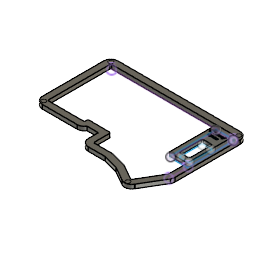
left_top_cover (Autodesk Fusion 360 design; units mm, degrees)
part number: 2026-07-17-00-49-13-895
Autodesk Fusion 360 part; units mm, degrees
note: some values were not read from the file. Set by a fixed rule: which sketch regions a step uses.
sketch "topcoverout1" plane through (0, 0, 0) normal (0, 0, 1) x (1, 0, 0)
  arc A0 (-38.1199, -35.6191) -> (-38.1206, -35.6555) centre (-37.1206, -35.6574) ccw
  line L0 (-38.1206, -35.6555) -> (-38.1199, -35.2716)
  line L1 (-38.1199, -35.2716) -> (-38.1199, -35.6191)
  line L2 (-63.0386, 17.2914) -> (-60.9186, 17.2914)
  line L3 (-72.6386, 3.6665) -> (-74.7361, 3.6665)
  line L4 (-60.941, 3.6665) -> (-63.0386, 3.6665)
  line L5 (-60.9226, 17.2877) -> (-60.9226, 13.2151)
  line L6 (-60.9226, 7.4151) -> (-60.9226, 3.6437)
  line L7 (-74.7546, 3.6437) -> (-74.7546, 7.4151)
  line L8 (-60.8212, 3.327) -> (-74.8212, 3.327)
  line L9 (-60.8212, 17.327) -> (-60.8212, 3.327)
  line L10 (-74.8212, 17.327) -> (-60.8212, 17.327)
  line L11 (-74.8212, 3.327) -> (-74.8212, 17.327)
  line L12 (-74.8212, 17.327) -> (-60.8212, 17.327)
  line L13 (-74.8212, 3.327) -> (-74.8212, 17.327)
  line L14 (-60.8681, -1.6074) -> (-60.8681, -15.6074)
  line L15 (-74.8681, -1.6074) -> (-60.8681, -1.6074)
  line L16 (-60.8681, -15.6074) -> (-74.8681, -15.6074)
  line L17 (-74.8681, -15.6074) -> (-74.8681, -1.6074)
  line L18 (-60.8756, -20.5875) -> (-60.8756, -34.5875)
  line L19 (-74.8756, -20.5875) -> (-60.8756, -20.5875)
  line L20 (-60.8756, -34.5875) -> (-74.8756, -34.5875)
  line L21 (-74.8756, -34.5875) -> (-74.8756, -20.5875)
  line L22 (-74.8618, 3.6522) -> (-74.8618, 17.6522)
  line L23 (-41.7744, 17.3824) -> (-41.7744, 3.3824)
  line L24 (-55.7744, 17.3824) -> (-41.7744, 17.3824)
  line L25 (-41.7744, 3.3824) -> (-55.7744, 3.3824)
  line L26 (-55.7744, 3.3824) -> (-55.7744, 17.3824)
  line L27 (-41.7619, -1.6704) -> (-41.7619, -15.6704)
  line L28 (-55.7619, -1.6704) -> (-41.7619, -1.6704)
  line L29 (-41.7619, -15.6704) -> (-55.7619, -15.6704)
  line L30 (-55.7619, -15.6704) -> (-55.7619, -1.6704)
  line L31 (-41.7679, -20.6705) -> (-41.7679, -34.6705)
  line L32 (-55.7679, -20.6705) -> (-41.7679, -20.6705)
  line L33 (-41.7679, -34.6705) -> (-55.7679, -34.6705)
  line L34 (-55.7679, -34.6705) -> (-55.7679, -20.6705)
  line L35 (-22.6973, 21.268) -> (-22.6973, 7.268)
  line L36 (-36.6973, 21.268) -> (-22.6973, 21.268)
  line L37 (-22.6973, 7.268) -> (-36.6973, 7.268)
  line L38 (-36.6973, 7.268) -> (-36.6973, 21.268)
  line L39 (-22.6915, 2.1961) -> (-22.6915, -11.8039)
  line L40 (-36.6915, 2.1961) -> (-22.6915, 2.1961)
  line L41 (-22.6915, -11.8039) -> (-36.6915, -11.8039)
  line L42 (-36.6915, -11.8039) -> (-36.6915, 2.1961)
  line L43 (44.6185, 10.2372) -> (44.6185, -15.5628)
  line L44 (55.9185, 10.2372) -> (44.6185, 10.2372)
  line L45 (44.6185, -15.5628) -> (55.9185, -15.5628)
  line L46 (55.9185, -15.5628) -> (55.9185, 10.2372)
  line L47 (-22.7318, -16.9097) -> (-22.7318, -30.9097)
  line L48 (-36.7318, -16.9097) -> (-22.7318, -16.9097)
  line L49 (-22.7318, -30.9097) -> (-36.7318, -30.9097)
  line L50 (-36.7318, -30.9097) -> (-36.7318, -16.9097)
  line L51 (-3.7525, 23.0596) -> (-3.7525, 9.0596)
  line L52 (-17.7525, 23.0596) -> (-3.7525, 23.0596)
  line L53 (-3.7525, 9.0596) -> (-17.7525, 9.0596)
  line L54 (-17.7525, 9.0596) -> (-17.7525, 23.0596)
  line L55 (-3.7007, 3.9637) -> (-3.7007, -10.0363)
  line L56 (-17.7007, 3.9637) -> (-3.7007, 3.9637)
  line L57 (-3.7007, -10.0363) -> (-17.7007, -10.0363)
  line L58 (-17.7007, -10.0363) -> (-17.7007, 3.9637)
  line L59 (-3.7688, -15.0165) -> (-3.7688, -29.0165)
  line L60 (-17.7688, -15.0165) -> (-3.7688, -15.0165)
  line L61 (-3.7688, -29.0165) -> (-17.7688, -29.0165)
  line L62 (-17.7688, -29.0165) -> (-17.7688, -15.0165)
  line L63 (15.4185, 21.139) -> (15.4185, 7.139)
  line L64 (1.4185, 21.139) -> (15.4185, 21.139)
  line L65 (15.4185, 7.139) -> (1.4185, 7.139)
  line L66 (1.4185, 7.139) -> (1.4185, 21.139)
  line L67 (15.4509, 2.0912) -> (15.4509, -11.9088)
  line L68 (1.4509, 2.0912) -> (15.4509, 2.0912)
  line L69 (15.4509, -11.9088) -> (1.4509, -11.9088)
  line L70 (1.4509, -11.9088) -> (1.4509, 2.0912)
  line L71 (15.4192, -16.9262) -> (15.4192, -30.9262)
  line L72 (1.4192, -16.9262) -> (15.4192, -16.9262)
  line L73 (15.4192, -30.9262) -> (1.4192, -30.9262)
  line L74 (1.4192, -30.9262) -> (1.4192, -16.9262)
  line L75 (34.4618, 19.276) -> (34.4618, 5.276)
  line L76 (20.4618, 19.276) -> (34.4618, 19.276)
  line L77 (34.4618, 5.276) -> (20.4618, 5.276)
  line L78 (20.4618, 5.276) -> (20.4618, 19.276)
  line L79 (34.3662, 0.0812) -> (34.3662, -13.9188)
  line L80 (20.3662, 0.0812) -> (34.3662, 0.0812)
  line L81 (34.3662, -13.9188) -> (20.3662, -13.9188)
  line L82 (20.3662, -13.9188) -> (20.3662, 0.0812)
  line L83 (34.4383, -18.8384) -> (34.4383, -32.8384)
  line L84 (20.4383, -18.8384) -> (34.4383, -18.8384)
  line L85 (34.4383, -32.8384) -> (20.4383, -32.8384)
  line L86 (20.4383, -32.8384) -> (20.4383, -18.8384)
  line L87 (5.8139, -35.9431) -> (5.8139, -49.9431)
  line L88 (-8.1861, -35.9431) -> (5.8139, -35.9431)
  line L89 (5.8139, -49.9431) -> (-8.1861, -49.9431)
  line L90 (-8.1861, -49.9431) -> (-8.1861, -35.9431)
  line L91 (28.7862, -40.8277) -> (25.1627, -54.3507)
  line L92 (15.2632, -37.2043) -> (28.7862, -40.8277)
  line L93 (25.1627, -54.3507) -> (11.6397, -50.7272)
  line L94 (11.6397, -50.7272) -> (15.2632, -37.2043)
  line L95 (51.7903, -47.2432) -> (44.7903, -59.3676)
  line L96 (39.666, -40.2432) -> (51.7903, -47.2432)
  line L97 (44.7903, -59.3676) -> (32.666, -52.3676)
  line L98 (32.666, -52.3676) -> (39.666, -40.2432)
  line L99 (39.9616, -20.2716) -> (39.9616, 29.8284)
  line L100 (39.9616, 29.8284) -> (59.3616, 29.8284)
  line L101 (59.3616, -20.2716) -> (39.9616, -20.2716)
  line L102 (59.3616, 29.8284) -> (59.3616, -20.2716)
  circle A1 centre (-81.2782, 34.061) radius 1.6
  circle A2 centre (-81.0384, -41.2716) radius 1.6
  circle A3 centre (43.9616, -72.2716) radius 1.6
  circle A4 centre (61.4616, 34.2284) radius 1.6
  line L103 (-37.1187, -34.6575) -> (-37.1033, -34.6575)
  line L104 (-37.1033, -34.6575) -> (-13.5537, -34.8219)
  arc A5 (-12.5607, -35.8288) -> (-13.5537, -34.8219) centre (-13.5606, -35.8219) ccw
  line L105 (-12.5607, -35.8288) -> (-12.5617, -35.9723)
  line L106 (-12.5617, -35.9723) -> (-12.558, -53.0098)
  arc A6 (-12.558, -53.0098) -> (-11.558, -54.0096) centre (-11.558, -53.0096) ccw
  line L107 (-11.558, -54.0096) -> (8.2128, -54.0096)
  arc A7 (8.4715, -54.0436) -> (8.2128, -54.0096) centre (8.2128, -55.0096) ccw
  line L108 (8.4715, -54.0436) -> (26.4518, -58.8585)
  arc A8 (26.6903, -58.9568) -> (26.4518, -58.8585) centre (26.1932, -59.8244) ccw
  line L109 (26.6903, -58.9568) -> (43.1014, -68.3607)
  arc A9 (43.1014, -68.3607) -> (44.4663, -67.9902) centre (43.5986, -67.4931) ccw
  line L110 (44.4663, -67.9902) -> (44.7236, -67.5412)
  line L111 (44.7236, -67.5412) -> (59.4411, -42.5979)
  arc A10 (59.4411, -42.5979) -> (59.5798, -42.0897) centre (58.5798, -42.0897) ccw
  line L112 (59.5798, -42.0897) -> (59.5798, 30.7287)
  arc A11 (59.5798, 30.7287) -> (58.5802, 31.7287) centre (58.5798, 30.7287) ccw
  line L113 (58.5802, 31.7287) -> (-78.1023, 31.7808)
  arc A12 (-78.1023, 31.7808) -> (-79.1027, 30.7808) centre (-78.1027, 30.7808) ccw
  line L114 (-79.1027, 30.7808) -> (-79.1027, -37.7188)
  arc A13 (-79.1027, -37.7188) -> (-78.1027, -38.7188) centre (-78.1027, -37.7188) ccw
  line L115 (-78.1027, -38.7188) -> (-39.1199, -38.7188)
  arc A14 (-39.1199, -38.7188) -> (-38.1199, -37.7188) centre (-39.1199, -37.7188) ccw
  line L116 (-38.1199, -37.7188) -> (-38.1199, -35.6191)
  arc A15 (-37.1187, -34.6575) -> (-38.1199, -35.6191) centre (-37.1206, -35.6574) ccw
  arc A16 (-19.558, -53.0113) -> (-11.558, -61.0096) centre (-11.558, -53.0096) ccw
  line L117 (-19.5604, -41.7801) -> (-19.558, -53.0113)
  line L118 (-86.1027, 30.7808) -> (-86.1027, 27.7812)
  arc A17 (65.4699, -46.1551) -> (66.5798, -42.0897) centre (58.5798, -42.0897) ccw
  line L119 (-7.292, -61.0096) -> (7.4234, -61.0096)
  arc A18 (-86.1027, -37.7188) -> (-78.1027, -45.7188) centre (-78.1027, -37.7188) ccw
  arc A19 (66.5798, 30.7287) -> (58.5829, 38.7287) centre (58.5798, 30.7287) ccw
  line L120 (50.775, -71.06) -> (53.5624, -66.336)
  line L121 (-32.1763, -41.692) -> (-19.5604, -41.7801)
  line L122 (-71.0384, -45.7188) -> (-39.1199, -45.7188)
  arc A20 (39.6212, -74.4342) -> (50.5398, -71.4705) centre (43.5986, -67.4931) ccw
  line L123 (-78.1027, -45.7188) -> (-71.0384, -45.7188)
  line L124 (7.4234, -61.0096) -> (23.8872, -65.4183)
  line L125 (50.5398, -71.4705) -> (50.775, -71.06)
  line L126 (39.4454, -74.3335) -> (39.6212, -74.4342)
  line L127 (58.5829, 38.7287) -> (-78.0996, 38.7808)
  line L128 (23.8872, -65.4183) -> (39.4454, -74.3335)
  arc A21 (-39.1199, -45.7188) -> (-32.1763, -41.692) centre (-39.1199, -37.7188) ccw
  line L129 (53.5624, -66.336) -> (58.9899, -57.1374)
  line L130 (66.5798, -42.0897) -> (66.5798, 30.7287)
  line L131 (-11.558, -61.0096) -> (-7.292, -61.0096)
  line L132 (58.9899, -57.1374) -> (64.9753, -46.9933)
  line L133 (-86.1027, 27.7812) -> (-86.1027, -37.7188)
  line L134 (64.9753, -46.9933) -> (65.4699, -46.1551)
  arc A22 (-78.0996, 38.7808) -> (-86.1027, 30.7808) centre (-78.1027, 30.7808) ccw
  point P0 (61.4616, 34.2284)
  point P1 (-81.2782, 34.061)
  point P2 (-81.0384, -41.2716)
  point P3 (43.9616, -72.2716)
sketch "Sketch2" plane through (0, 0, 0) normal (0, 0, 1) x (1, 0, 0)
  line L0 (39.9616, 29.8284) -> (59.3616, 29.8284)
  line L1 (39.9616, -20.2716) -> (39.9616, 29.8284)
  line L2 (59.3616, -20.2716) -> (39.9616, -20.2716)
  line L3 (58.5802, 31.7287) -> (-78.1023, 31.7808)
  arc A0 (59.5798, 30.7287) -> (58.5802, 31.7287) centre (58.5798, 30.7287) ccw
  line L4 (59.5798, -42.0897) -> (59.5798, 30.7287)
  line L5 (38.6875, 31.7363) -> (58.5798, 31.7363)
  line L6 (59.5798, 30.7363) -> (59.5798, -21.2716)
  line L7 (59.5798, -21.2716) -> (39.6875, -21.2716)
  line L8 (38.6875, -20.2716) -> (38.6875, 31.7363)
  arc A1 (59.5798, 30.7363) -> (58.5798, 31.7363) centre (58.5798, 30.7363) ccw
  arc A2 (38.6875, -20.2716) -> (39.6875, -21.2716) centre (39.6875, -20.2716) ccw
  line L9 (45.6185, 10.2372) -> (54.9185, 10.2372)
  line L10 (55.9185, 9.2372) -> (55.9185, -14.5628)
  line L11 (54.9185, -15.5628) -> (45.6185, -15.5628)
  line L12 (44.6185, -14.5628) -> (44.6185, 9.2372)
  arc A3 (45.6185, 10.2372) -> (44.6185, 9.2372) centre (45.6185, 9.2372) ccw
  arc A4 (55.9185, 9.2372) -> (54.9185, 10.2372) centre (54.9185, 9.2372) ccw
  arc A5 (54.9185, -15.5628) -> (55.9185, -14.5628) centre (54.9185, -14.5628) ccw
  arc A6 (44.6185, -14.5628) -> (45.6185, -15.5628) centre (45.6185, -14.5628) ccw
  dimension "d3" = 1
  dimension "d4" = 1
  dimension "d5" = 1
  constraint perpendicular L5 L6
  constraint parallel L5 L7
  constraint parallel L6 L8
  constraint perpendicular L4 L5
  constraint coincident L3 L5.start
  constraint tangent L5 A1
  constraint tangent L6 A1
  constraint tangent L7 A2
  constraint tangent L8 A2
  constraint perpendicular L9 L10
  constraint parallel L9 L11
  constraint parallel L10 L12
  constraint tangent L9 A3
  constraint tangent L12 A3
  constraint tangent L9 A4
  constraint tangent L10 A4
  constraint equal A3 A4
  constraint tangent L10 A5
  constraint tangent L11 A5
  constraint equal A3 A5
  constraint tangent L11 A6
  constraint tangent L12 A6
  constraint equal A3 A6
  measures "d3" radius of A1
  measures "d4" radius of A2
  measures "d5" radius of A3
extrude "Extrude1" add sketch "topcoverout1" along normal blind 4.5 contours A1 | A2 | A3 | A4 | A16 L117 L118 A17 L119 A18 A19 L120 L121 L122 A20 L123 L124 L125 L126 L127 L128 A21 L129 L130 L131 L132 L133 L134 A22 picked at (-81.0115, 33.1363) picked at (-80.7717, -42.1963) picked at (43.6291, -73.003) picked at (61.7283, 35.0046) picked at (13.0203, 34.0794) makes body 1
extrude "Extrude2" add sketch "Sketch2" along normal blind 4.5 separate body contours L3 A0 L4 L6 L7 L8 A2 picked at (47.6287, 24.5674) makes body 2
sketch "Sketch3" plane through (0, 0, 0) normal (0, 0, 1) x (1, 0, 0)
  circle A0 centre (61.4616, 34.2284) radius 1.6
  circle A1 centre (43.9616, -72.2716) radius 1.6
  circle A2 centre (-81.2782, 34.061) radius 1.6
  circle A3 centre (61.4616, 34.2284) radius 2.45
  circle A4 centre (43.9616, -72.2716) radius 2.45
  circle A5 centre (-81.0384, -41.2716) radius 2.45
  circle A6 centre (-81.2782, 34.061) radius 2.45
  point P0 (-81.0384, -41.2716)
  dimension "d8" = 4.9
  dimension "d9" = 4.9
  dimension "d10" = 4.9
  dimension "d11" = 4.9
  constraint concentric A0 A3
  constraint concentric A1 A4
  constraint coincident P0 A5.centre
  constraint concentric A2 A6
  measures "d8" diameter of A3
  measures "d9" diameter of A4
  measures "d10" diameter of A5
  measures "d11" diameter of A6
extrude "Extrude3" cut sketch "Sketch3" along normal blind 3.9 contours A0 | A1 | A2 | A3 | A4 | A6 picked at (61.7283, 35.0046) picked at (43.6291, -73.003) picked at (-81.0115, 33.1363) picked at (59.3463, 34.6703) picked at (45.8128, -73.3865) picked at (-80.9955, 36.2034) bodies 1
extrude "Extrude4" cut sketch "Sketch3" along normal blind 3.9 contours A5 picked at (-79.2238, -40.9981) bodies 1
extrude "Extrude5" cut 1 faces at (47.6287, 24.5674, 0) along direction (0, 0, 1) blind 0.5 on bodies 2 bodies 2
extrude "Extrude6" cut 1 faces at (47.6287, 24.5674, 0.5) along direction (0, 0, 1) blind 0.5 on bodies 2 bodies 2
sketch "Sketch4" plane through (0, 0, 4.5) normal (0, 0, 1) x (-1, 0, 0)
  arc A0 (-45.6185, -10.2372) -> (-44.6185, -9.2372) centre (-45.6185, -9.2372) ccw
  line L0 (-45.6185, -10.2372) -> (-54.9185, -10.2372)
  arc A1 (-55.9185, -9.2372) -> (-54.9185, -10.2372) centre (-54.9185, -9.2372) ccw
  line L1 (-55.9185, -9.2372) -> (-55.9185, 14.5628)
  arc A2 (-54.9185, 15.5628) -> (-55.9185, 14.5628) centre (-54.9185, 14.5628) ccw
  line L2 (-54.9185, 15.5628) -> (-45.6185, 15.5628)
  arc A3 (-44.6185, 14.5628) -> (-45.6185, 15.5628) centre (-45.6185, 14.5628) ccw
  line L3 (-44.6185, 14.5628) -> (-44.6185, -9.2372)
  arc A4 (-59.5798, -30.7287) -> (-58.5802, -31.7287) centre (-58.5798, -30.7287) ccw
  line L4 (-58.5802, -31.7287) -> (-38.6875, -31.7363)
  line L5 (-38.6875, -31.7363) -> (-38.6875, 20.2716)
  arc A5 (-38.6875, 20.2716) -> (-39.6875, 21.2716) centre (-39.6875, 20.2716) ccw
  line L6 (-39.6875, 21.2716) -> (-59.5798, 21.2716)
  line L7 (-59.5798, 21.2716) -> (-59.5798, -30.7287)
  spline S0 degree 2 poles (-41.2211, -21.734) (-40.7461, -21.7358) (-40.5191, -21.9812) knots 0 0 0 1 1 1
  spline S1 degree 2 poles (-40.5191, -21.9812) (-40.2922, -22.2266) (-40.2904, -22.7615) knots 0 0 0 1 1 1
  spline S2 degree 2 poles (-40.2904, -22.7615) (-40.2922, -23.1837) (-40.3872, -23.5435) knots 0 0 0 1 1 1
  spline S3 degree 2 poles (-40.3872, -23.5435) (-40.4822, -23.9033) (-40.6564, -24.1707) knots 0 0 0 1 1 1
  spline S4 degree 2 poles (-40.6564, -24.1707) (-40.8305, -24.4381) (-41.0628, -24.5868) knots 0 0 0 1 1 1
  spline S5 degree 2 poles (-41.0628, -24.5868) (-41.295, -24.7354) (-41.5677, -24.7354) knots 0 0 0 1 1 1
  spline S6 degree 2 poles (-41.5677, -24.7354) (-42.2046, -24.7354) (-42.2046, -24.0827) knots 0 0 0 1 1 1
  spline S7 degree 2 poles (-42.2046, -24.0827) (-42.2063, -23.9807) (-42.1703, -23.766) knots 0 0 0 1 1 1
  spline S8 degree 2 poles (-42.1703, -23.766) (-42.1342, -23.5514) (-42.0585, -23.1256) knots 0 0 0 1 1 1
  line L8 (-42.0585, -23.1256) -> (-41.6891, -23.1256)
  spline S9 degree 2 poles (-41.6891, -23.1256) (-41.7295, -23.3667) (-41.7542, -23.5215) knots 0 0 0 1 1 1
  spline S10 degree 2 poles (-41.7542, -23.5215) (-41.7788, -23.6763) (-41.7911, -23.7678) knots 0 0 0 1 1 1
  spline S11 degree 2 poles (-41.7911, -23.7678) (-41.8034, -23.8593) (-41.8096, -23.9112) knots 0 0 0 1 1 1
  spline S12 degree 2 poles (-41.8096, -23.9112) (-41.8158, -23.9631) (-41.8228, -23.9965) knots 0 0 0 1 1 1
  spline S13 degree 2 poles (-41.8228, -23.9965) (-41.8245, -24.2094) (-41.7463, -24.2824) knots 0 0 0 1 1 1
  spline S14 degree 2 poles (-41.7463, -24.2824) (-41.668, -24.3554) (-41.5149, -24.3554) knots 0 0 0 1 1 1
  spline S15 degree 2 poles (-41.5149, -24.3554) (-41.3407, -24.3572) (-41.1877, -24.2323) knots 0 0 0 1 1 1
  spline S16 degree 2 poles (-41.1877, -24.2323) (-41.0346, -24.1073) (-40.9176, -23.8892) knots 0 0 0 1 1 1
  spline S17 degree 2 poles (-40.9176, -23.8892) (-40.8006, -23.671) (-40.7338, -23.3843) knots 0 0 0 1 1 1
  spline S18 degree 2 poles (-40.7338, -23.3843) (-40.6669, -23.0975) (-40.6687, -22.772) knots 0 0 0 1 1 1
  spline S19 degree 2 poles (-40.6687, -22.772) (-40.6687, -22.4307) (-40.805, -22.2715) knots 0 0 0 1 1 1
  spline S20 degree 2 poles (-40.805, -22.2715) (-40.9414, -22.1123) (-41.2246, -22.114) knots 0 0 0 1 1 1
  spline S21 degree 2 poles (-41.2246, -22.114) (-41.4498, -22.114) (-41.587, -22.1562) knots 0 0 0 1 1 1
  line L9 (-41.587, -22.1562) -> (-41.5343, -21.778)
  spline S22 degree 2 poles (-41.5343, -21.778) (-41.4023, -21.7358) (-41.2211, -21.734) knots 0 0 0 1 1 1
  spline S23 degree 2 poles (-41.2123, -22.4395) (-41.0557, -22.4395) (-40.9704, -22.5688) knots 0 0 0 1 1 1
  spline S24 degree 2 poles (-40.9704, -22.5688) (-40.8851, -22.6981) (-40.8851, -22.9304) knots 0 0 0 1 1 1
  spline S25 degree 2 poles (-40.8851, -22.9304) (-40.8851, -23.2646) (-41.0117, -23.5188) knots 0 0 0 1 1 1
  spline S26 degree 2 poles (-41.0117, -23.5188) (-41.1384, -23.7731) (-41.3592, -23.9296) knots 0 0 0 1 1 1
  spline S27 degree 2 poles (-41.3592, -23.9296) (-41.58, -24.0862) (-41.8615, -24.1214) knots 0 0 0 1 1 1
  line L10 (-41.8615, -24.1214) -> (-41.8386, -23.7396)
  spline S28 degree 2 poles (-41.8386, -23.7396) (-41.6715, -23.7326) (-41.5351, -23.635) knots 0 0 0 1 1 1
  spline S29 degree 2 poles (-41.5351, -23.635) (-41.3988, -23.5373) (-41.3196, -23.3755) knots 0 0 0 1 1 1
  spline S30 degree 2 poles (-41.3196, -23.3755) (-41.2405, -23.2136) (-41.2405, -23.0095) knots 0 0 0 1 1 1
  spline S31 degree 2 poles (-41.2405, -23.0095) (-41.2405, -22.9057) (-41.2774, -22.8529) knots 0 0 0 1 1 1
  spline S32 degree 2 poles (-41.2774, -22.8529) (-41.3143, -22.8002) (-41.3865, -22.8002) knots 0 0 0 1 1 1
  spline S33 degree 2 poles (-41.3865, -22.8002) (-41.4674, -22.8002) (-41.5307, -22.8609) knots 0 0 0 1 1 1
  spline S34 degree 2 poles (-41.5307, -22.8609) (-41.5941, -22.9216) (-41.6469, -23.0641) knots 0 0 0 1 1 1
  spline S35 degree 2 poles (-41.6469, -23.0641) (-41.6996, -23.2066) (-41.7454, -23.4529) knots 0 0 0 1 1 1
  line L11 (-41.7454, -23.4529) -> (-42.1166, -23.4529)
  line L12 (-42.1166, -23.4529) -> (-41.9442, -22.4729)
  line L13 (-41.9442, -22.4729) -> (-41.6152, -22.4729)
  line L14 (-41.6152, -22.4729) -> (-41.6697, -23.0236)
  line L15 (-41.6697, -23.0236) -> (-41.7718, -22.8477)
  line L16 (-41.7718, -22.8477) -> (-41.5765, -22.8459)
  line L17 (-41.5765, -22.8459) -> (-41.6398, -22.9409)
  spline S36 degree 2 poles (-41.6398, -22.9409) (-41.587, -22.7034) (-41.4736, -22.5723) knots 0 0 0 1 1 1
  spline S37 degree 2 poles (-41.4736, -22.5723) (-41.3601, -22.4413) (-41.2123, -22.4395) knots 0 0 0 1 1 1
  line L18 (-42.9452, -22.2037) -> (-43.1282, -23.2488)
  line L19 (-43.1282, -23.2488) -> (-43.5575, -23.2488)
  line L20 (-43.5575, -23.2488) -> (-43.3745, -22.2037)
  line L21 (-43.3745, -22.2037) -> (-42.9452, -22.2037)
  line L22 (-43.1106, -22.9708) -> (-42.5652, -24.6633)
  line L23 (-42.5652, -24.6633) -> (-43.0015, -24.7196)
  line L24 (-43.0015, -24.7196) -> (-43.3675, -23.4071)
  line L25 (-43.3675, -23.4071) -> (-43.3991, -23.4071)
  spline S38 degree 2 poles (-43.3991, -23.4071) (-43.5856, -23.6024) (-43.7281, -23.7933) knots 0 0 0 1 1 1
  spline S39 degree 2 poles (-43.7281, -23.7933) (-43.8706, -23.9842) (-43.9815, -24.2032) knots 0 0 0 1 1 1
  spline S40 degree 2 poles (-43.9815, -24.2032) (-44.0923, -24.4223) (-44.1803, -24.702) knots 0 0 0 1 1 1
  line L26 (-44.1803, -24.702) -> (-44.6307, -24.702)
  spline S41 degree 2 poles (-44.6307, -24.702) (-44.5146, -24.329) (-44.3448, -24.0247) knots 0 0 0 1 1 1
  spline S42 degree 2 poles (-44.3448, -24.0247) (-44.175, -23.7203) (-43.9481, -23.4564) knots 0 0 0 1 1 1
  spline S43 degree 2 poles (-43.9481, -23.4564) (-43.7211, -23.1925) (-43.4326, -22.9321) knots 0 0 0 1 1 1
  line L27 (-43.4326, -22.9321) -> (-43.1106, -22.9708)
  spline S44 degree 2 poles (-45.264, -22.1686) (-44.9421, -22.1686) (-44.7626, -22.3471) knots 0 0 0 1 1 1
  spline S45 degree 2 poles (-44.7626, -22.3471) (-44.5832, -22.5257) (-44.5832, -22.8441) knots 0 0 0 1 1 1
  spline S46 degree 2 poles (-44.5832, -22.8441) (-44.5814, -23.4388) (-44.8523, -23.7713) knots 0 0 0 1 1 1
  spline S47 degree 2 poles (-44.8523, -23.7713) (-45.1233, -24.1038) (-45.6053, -24.1038) knots 0 0 0 1 1 1
  spline S48 degree 2 poles (-45.6053, -24.1038) (-45.9273, -24.1038) (-46.1067, -23.9208) knots 0 0 0 1 1 1
  spline S49 degree 2 poles (-46.1067, -23.9208) (-46.2862, -23.7379) (-46.2862, -23.4106) knots 0 0 0 1 1 1
  spline S50 degree 2 poles (-46.2862, -23.4106) (-46.288, -22.8248) (-46.017, -22.4967) knots 0 0 0 1 1 1
  spline S51 degree 2 poles (-46.017, -22.4967) (-45.7461, -22.1686) (-45.264, -22.1686) knots 0 0 0 1 1 1
  spline S52 degree 2 poles (-45.3397, -22.5714) (-45.5772, -22.5732) (-45.7109, -22.7747) knots 0 0 0 1 1 1
  spline S53 degree 2 poles (-45.7109, -22.7747) (-45.8446, -22.9761) (-45.8428, -23.335) knots 0 0 0 1 1 1
  spline S54 degree 2 poles (-45.8428, -23.335) (-45.8446, -23.5074) (-45.7646, -23.6033) knots 0 0 0 1 1 1
  spline S55 degree 2 poles (-45.7646, -23.6033) (-45.6845, -23.6992) (-45.5402, -23.6992) knots 0 0 0 1 1 1
  spline S56 degree 2 poles (-45.5402, -23.6992) (-45.2975, -23.6992) (-45.1611, -23.4986) knots 0 0 0 1 1 1
  spline S57 degree 2 poles (-45.1611, -23.4986) (-45.0248, -23.298) (-45.0265, -22.9374) knots 0 0 0 1 1 1
  spline S58 degree 2 poles (-45.0265, -22.9374) (-45.0248, -22.765) (-45.1083, -22.6682) knots 0 0 0 1 1 1
  spline S59 degree 2 poles (-45.1083, -22.6682) (-45.1919, -22.5714) (-45.3397, -22.5714) knots 0 0 0 1 1 1
  spline S60 degree 2 poles (-47.1729, -22.1668) (-46.9178, -22.1668) (-46.7788, -22.3251) knots 0 0 0 1 1 1
  spline S61 degree 2 poles (-46.7788, -22.3251) (-46.6398, -22.4835) (-46.6398, -22.7685) knots 0 0 0 1 1 1
  spline S62 degree 2 poles (-46.6398, -22.7685) (-46.6398, -23.0306) (-46.7243, -23.3464) knots 0 0 0 1 1 1
  spline S63 degree 2 poles (-46.7243, -23.3464) (-46.8087, -23.6622) (-46.997, -24.1038) knots 0 0 0 1 1 1
  line L28 (-46.997, -24.1038) -> (-47.4333, -24.0352)
  spline S64 degree 2 poles (-47.4333, -24.0352) (-47.2485, -23.5848) (-47.165, -23.2945) knots 0 0 0 1 1 1
  spline S65 degree 2 poles (-47.165, -23.2945) (-47.0814, -23.0042) (-47.0814, -22.8125) knots 0 0 0 1 1 1
  spline S66 degree 2 poles (-47.0814, -22.8125) (-47.0814, -22.6981) (-47.143, -22.6348) knots 0 0 0 1 1 1
  spline S67 degree 2 poles (-47.143, -22.6348) (-47.2046, -22.5714) (-47.3189, -22.5714) knots 0 0 0 1 1 1
  spline S68 degree 2 poles (-47.3189, -22.5714) (-47.5283, -22.5714) (-47.662, -22.779) knots 0 0 0 1 1 1
  spline S69 degree 2 poles (-47.662, -22.779) (-47.7957, -22.9866) (-47.8713, -23.3772) knots 0 0 0 1 1 1
  line L29 (-47.8713, -23.3772) -> (-47.8467, -22.6172)
  line L30 (-47.8467, -22.6172) -> (-47.7306, -22.6172)
  line L31 (-47.7306, -22.6172) -> (-47.8133, -22.7615)
  spline S70 degree 2 poles (-47.8133, -22.7615) (-47.7535, -22.5785) (-47.6822, -22.4448) knots 0 0 0 1 1 1
  spline S71 degree 2 poles (-47.6822, -22.4448) (-47.611, -22.3111) (-47.4922, -22.2389) knots 0 0 0 1 1 1
  spline S72 degree 2 poles (-47.4922, -22.2389) (-47.3735, -22.1668) (-47.1729, -22.1668) knots 0 0 0 1 1 1
  spline S73 degree 2 poles (-48.2496, -22.1862) (-48.0842, -22.1862) (-47.9839, -22.2372) knots 0 0 0 1 1 1
  spline S74 degree 2 poles (-47.9839, -22.2372) (-47.8837, -22.2882) (-47.8458, -22.3911) knots 0 0 0 1 1 1
  spline S75 degree 2 poles (-47.8458, -22.3911) (-47.808, -22.494) (-47.8291, -22.6541) knots 0 0 0 1 1 1
  line L32 (-47.8291, -22.6541) -> (-47.8133, -23.05)
  line L33 (-47.8133, -23.05) -> (-47.9945, -24.0686)
  line L34 (-47.9945, -24.0686) -> (-48.4361, -24.0686)
  line L35 (-48.4361, -24.0686) -> (-48.2127, -22.8019)
  spline S76 degree 2 poles (-48.2127, -22.8019) (-48.188, -22.6612) (-48.225, -22.6058) knots 0 0 0 1 1 1
  spline S77 degree 2 poles (-48.225, -22.6058) (-48.2619, -22.5503) (-48.3816, -22.5503) knots 0 0 0 1 1 1
  line L36 (-48.3816, -22.5503) -> (-48.4625, -22.5503)
  line L37 (-48.4625, -22.5503) -> (-48.3974, -22.1862)
  line L38 (-48.3974, -22.1862) -> (-48.2496, -22.1862)
  spline S78 degree 2 poles (-49.3932, -22.1686) (-49.1768, -22.1686) (-49.0017, -22.1879) knots 0 0 0 1 1 1
  spline S79 degree 2 poles (-49.0017, -22.1879) (-48.8267, -22.2073) (-48.7053, -22.2425) knots 0 0 0 1 1 1
  line L39 (-48.7053, -22.2425) -> (-48.8284, -22.6506)
  spline S80 degree 2 poles (-48.8284, -22.6506) (-49.0448, -22.6137) (-49.2067, -22.5934) knots 0 0 0 1 1 1
  spline S81 degree 2 poles (-49.2067, -22.5934) (-49.3685, -22.5732) (-49.4653, -22.5732) knots 0 0 0 1 1 1
  spline S82 degree 2 poles (-49.4653, -22.5732) (-49.701, -22.5732) (-49.8233, -22.6233) knots 0 0 0 1 1 1
  spline S83 degree 2 poles (-49.8233, -22.6233) (-49.9456, -22.6735) (-49.9456, -22.7703) knots 0 0 0 1 1 1
  spline S84 degree 2 poles (-49.9456, -22.7703) (-49.9456, -22.809) (-49.9139, -22.8371) knots 0 0 0 1 1 1
  spline S85 degree 2 poles (-49.9139, -22.8371) (-49.8823, -22.8653) (-49.8242, -22.8846) knots 0 0 0 1 1 1
  line L40 (-49.8242, -22.8846) -> (-49.226, -23.0729)
  spline S86 degree 2 poles (-49.226, -23.0729) (-49.0818, -23.1186) (-49.0096, -23.2127) knots 0 0 0 1 1 1
  spline S87 degree 2 poles (-49.0096, -23.2127) (-48.9375, -23.3068) (-48.9375, -23.437) knots 0 0 0 1 1 1
  spline S88 degree 2 poles (-48.9375, -23.437) (-48.9375, -23.766) (-49.2084, -23.9349) knots 0 0 0 1 1 1
  spline S89 degree 2 poles (-49.2084, -23.9349) (-49.4794, -24.1038) (-50.0054, -24.1038) knots 0 0 0 1 1 1
  spline S90 degree 2 poles (-50.0054, -24.1038) (-50.1409, -24.1038) (-50.2851, -24.0933) knots 0 0 0 1 1 1
  spline S91 degree 2 poles (-50.2851, -24.0933) (-50.4294, -24.0827) (-50.5719, -24.0616) knots 0 0 0 1 1 1
  line L41 (-50.5719, -24.0616) -> (-50.4576, -23.6675)
  spline S92 degree 2 poles (-50.4576, -23.6675) (-50.3027, -23.6816) (-50.169, -23.6904) knots 0 0 0 1 1 1
  spline S93 degree 2 poles (-50.169, -23.6904) (-50.0353, -23.6992) (-49.9298, -23.6992) knots 0 0 0 1 1 1
  spline S94 degree 2 poles (-49.9298, -23.6992) (-49.6641, -23.6992) (-49.5278, -23.6482) knots 0 0 0 1 1 1
  spline S95 degree 2 poles (-49.5278, -23.6482) (-49.3914, -23.5971) (-49.3914, -23.5004) knots 0 0 0 1 1 1
  spline S96 degree 2 poles (-49.3914, -23.5004) (-49.3914, -23.4669) (-49.4187, -23.4432) knots 0 0 0 1 1 1
  spline S97 degree 2 poles (-49.4187, -23.4432) (-49.4459, -23.4194) (-49.497, -23.4054) knots 0 0 0 1 1 1
  line L42 (-49.497, -23.4054) -> (-50.0107, -23.2505)
  spline S98 degree 2 poles (-50.0107, -23.2505) (-50.206, -23.1907) (-50.3071, -23.0781) knots 0 0 0 1 1 1
  spline S99 degree 2 poles (-50.3071, -23.0781) (-50.4083, -22.9655) (-50.4083, -22.8072) knots 0 0 0 1 1 1
  spline S100 degree 2 poles (-50.4083, -22.8072) (-50.4083, -22.494) (-50.1506, -22.3313) knots 0 0 0 1 1 1
  spline S101 degree 2 poles (-50.1506, -22.3313) (-49.8928, -22.1686) (-49.3932, -22.1686) knots 0 0 0 1 1 1
  spline S102 degree 2 poles (-51.5044, -22.1686) (-51.288, -22.1686) (-51.1129, -22.1879) knots 0 0 0 1 1 1
  spline S103 degree 2 poles (-51.1129, -22.1879) (-50.9378, -22.2073) (-50.8165, -22.2425) knots 0 0 0 1 1 1
  line L43 (-50.8165, -22.2425) -> (-50.9396, -22.6506)
  spline S104 degree 2 poles (-50.9396, -22.6506) (-51.156, -22.6137) (-51.3179, -22.5934) knots 0 0 0 1 1 1
  spline S105 degree 2 poles (-51.3179, -22.5934) (-51.4797, -22.5732) (-51.5765, -22.5732) knots 0 0 0 1 1 1
  spline S106 degree 2 poles (-51.5765, -22.5732) (-51.8122, -22.5732) (-51.9345, -22.6233) knots 0 0 0 1 1 1
  spline S107 degree 2 poles (-51.9345, -22.6233) (-52.0568, -22.6735) (-52.0568, -22.7703) knots 0 0 0 1 1 1
  spline S108 degree 2 poles (-52.0568, -22.7703) (-52.0568, -22.809) (-52.0251, -22.8371) knots 0 0 0 1 1 1
  spline S109 degree 2 poles (-52.0251, -22.8371) (-51.9934, -22.8653) (-51.9354, -22.8846) knots 0 0 0 1 1 1
  line L44 (-51.9354, -22.8846) -> (-51.3372, -23.0729)
  spline S110 degree 2 poles (-51.3372, -23.0729) (-51.193, -23.1186) (-51.1208, -23.2127) knots 0 0 0 1 1 1
  spline S111 degree 2 poles (-51.1208, -23.2127) (-51.0487, -23.3068) (-51.0487, -23.437) knots 0 0 0 1 1 1
  spline S112 degree 2 poles (-51.0487, -23.437) (-51.0487, -23.766) (-51.3196, -23.9349) knots 0 0 0 1 1 1
  spline S113 degree 2 poles (-51.3196, -23.9349) (-51.5906, -24.1038) (-52.1166, -24.1038) knots 0 0 0 1 1 1
  spline S114 degree 2 poles (-52.1166, -24.1038) (-52.2521, -24.1038) (-52.3963, -24.0933) knots 0 0 0 1 1 1
  spline S115 degree 2 poles (-52.3963, -24.0933) (-52.5406, -24.0827) (-52.6831, -24.0616) knots 0 0 0 1 1 1
  line L45 (-52.6831, -24.0616) -> (-52.5687, -23.6675)
  spline S116 degree 2 poles (-52.5687, -23.6675) (-52.4139, -23.6816) (-52.2802, -23.6904) knots 0 0 0 1 1 1
  spline S117 degree 2 poles (-52.2802, -23.6904) (-52.1465, -23.6992) (-52.0409, -23.6992) knots 0 0 0 1 1 1
  spline S118 degree 2 poles (-52.0409, -23.6992) (-51.7753, -23.6992) (-51.6389, -23.6482) knots 0 0 0 1 1 1
  spline S119 degree 2 poles (-51.6389, -23.6482) (-51.5026, -23.5971) (-51.5026, -23.5004) knots 0 0 0 1 1 1
  spline S120 degree 2 poles (-51.5026, -23.5004) (-51.5026, -23.4669) (-51.5299, -23.4432) knots 0 0 0 1 1 1
  spline S121 degree 2 poles (-51.5299, -23.4432) (-51.5571, -23.4194) (-51.6082, -23.4054) knots 0 0 0 1 1 1
  line L46 (-51.6082, -23.4054) -> (-52.1219, -23.2505)
  spline S122 degree 2 poles (-52.1219, -23.2505) (-52.3172, -23.1907) (-52.4183, -23.0781) knots 0 0 0 1 1 1
  spline S123 degree 2 poles (-52.4183, -23.0781) (-52.5195, -22.9655) (-52.5195, -22.8072) knots 0 0 0 1 1 1
  spline S124 degree 2 poles (-52.5195, -22.8072) (-52.5195, -22.494) (-52.2617, -22.3313) knots 0 0 0 1 1 1
  spline S125 degree 2 poles (-52.2617, -22.3313) (-52.004, -22.1686) (-51.5044, -22.1686) knots 0 0 0 1 1 1
  spline S126 degree 2 poles (-53.8918, -22.5732) (-54.0219, -22.5732) (-54.1732, -22.6137) knots 0 0 0 1 1 1
  spline S127 degree 2 poles (-54.1732, -22.6137) (-54.3245, -22.6541) (-54.4635, -22.7298) knots 0 0 0 1 1 1
  line L47 (-54.4635, -22.7298) -> (-54.5849, -22.3586)
  spline S128 degree 2 poles (-54.5849, -22.3586) (-54.416, -22.2618) (-54.2225, -22.2152) knots 0 0 0 1 1 1
  spline S129 degree 2 poles (-54.2225, -22.2152) (-54.029, -22.1686) (-53.8548, -22.1686) knots 0 0 0 1 1 1
  spline S130 degree 2 poles (-53.8548, -22.1686) (-53.4783, -22.1686) (-53.2663, -22.3638) knots 0 0 0 1 1 1
  spline S131 degree 2 poles (-53.2663, -22.3638) (-53.0543, -22.5591) (-53.0543, -22.9092) knots 0 0 0 1 1 1
  spline S132 degree 2 poles (-53.0543, -22.9092) (-53.0543, -23.2681) (-53.1951, -23.5364) knots 0 0 0 1 1 1
  spline S133 degree 2 poles (-53.1951, -23.5364) (-53.3358, -23.8047) (-53.5892, -23.9543) knots 0 0 0 1 1 1
  spline S134 degree 2 poles (-53.5892, -23.9543) (-53.8425, -24.1038) (-54.1785, -24.1038) knots 0 0 0 1 1 1
  spline S135 degree 2 poles (-54.1785, -24.1038) (-54.4547, -24.1038) (-54.6104, -23.9657) knots 0 0 0 1 1 1
  spline S136 degree 2 poles (-54.6104, -23.9657) (-54.7661, -23.8276) (-54.7661, -23.5795) knots 0 0 0 1 1 1
  spline S137 degree 2 poles (-54.7661, -23.5795) (-54.7661, -23.2382) (-54.416, -23.0632) knots 0 0 0 1 1 1
  spline S138 degree 2 poles (-54.416, -23.0632) (-54.0659, -22.8881) (-53.4132, -22.8776) knots 0 0 0 1 1 1
  line L48 (-53.4132, -22.8776) -> (-53.3552, -23.1907)
  spline S139 degree 2 poles (-53.3552, -23.1907) (-53.8179, -23.196) (-54.0756, -23.2901) knots 0 0 0 1 1 1
  spline S140 degree 2 poles (-54.0756, -23.2901) (-54.3333, -23.3843) (-54.3333, -23.5479) knots 0 0 0 1 1 1
  spline S141 degree 2 poles (-54.3333, -23.5479) (-54.3351, -23.6235) (-54.2762, -23.6666) knots 0 0 0 1 1 1
  spline S142 degree 2 poles (-54.2762, -23.6666) (-54.2172, -23.7097) (-54.1082, -23.708) knots 0 0 0 1 1 1
  spline S143 degree 2 poles (-54.1082, -23.708) (-53.9164, -23.7097) (-53.7695, -23.6147) knots 0 0 0 1 1 1
  spline S144 degree 2 poles (-53.7695, -23.6147) (-53.6226, -23.5197) (-53.5416, -23.3491) knots 0 0 0 1 1 1
  spline S145 degree 2 poles (-53.5416, -23.3491) (-53.4607, -23.1784) (-53.459, -22.9515) knots 0 0 0 1 1 1
  spline S146 degree 2 poles (-53.459, -22.9515) (-53.459, -22.772) (-53.5733, -22.6726) knots 0 0 0 1 1 1
  spline S147 degree 2 poles (-53.5733, -22.6726) (-53.6877, -22.5732) (-53.8918, -22.5732) knots 0 0 0 1 1 1
  line L49 (-54.8084, -21.3681) -> (-54.7943, -21.771)
  line L50 (-54.7943, -21.771) -> (-54.9931, -21.7921)
  spline S148 degree 2 poles (-54.9931, -21.7921) (-55.1743, -21.8132) (-55.2992, -21.8836) knots 0 0 0 1 1 1
  spline S149 degree 2 poles (-55.2992, -21.8836) (-55.4241, -21.9539) (-55.4954, -22.0894) knots 0 0 0 1 1 1
  spline S150 degree 2 poles (-55.4954, -22.0894) (-55.5666, -22.2249) (-55.5842, -22.436) knots 0 0 0 1 1 1
  line L51 (-55.5842, -22.436) -> (-55.732, -23.8399)
  spline S151 degree 2 poles (-55.732, -23.8399) (-55.7654, -24.2023) (-55.8983, -24.4319) knots 0 0 0 1 1 1
  spline S152 degree 2 poles (-55.8983, -24.4319) (-56.0311, -24.6615) (-56.2721, -24.7697) knots 0 0 0 1 1 1
  spline S153 degree 2 poles (-56.2721, -24.7697) (-56.5131, -24.8779) (-56.8703, -24.8779) knots 0 0 0 1 1 1
  spline S154 degree 2 poles (-56.8703, -24.8779) (-57.0621, -24.8779) (-57.2327, -24.8427) knots 0 0 0 1 1 1
  line L52 (-57.2327, -24.8427) -> (-57.1219, -24.4486)
  spline S155 degree 2 poles (-57.1219, -24.4486) (-57.0146, -24.4627) (-56.9363, -24.468) knots 0 0 0 1 1 1
  spline S156 degree 2 poles (-56.9363, -24.468) (-56.858, -24.4733) (-56.7894, -24.4733) knots 0 0 0 1 1 1
  spline S157 degree 2 poles (-56.7894, -24.4733) (-56.4991, -24.4733) (-56.3513, -24.3264) knots 0 0 0 1 1 1
  spline S158 degree 2 poles (-56.3513, -24.3264) (-56.2035, -24.1795) (-56.1718, -23.8575) knots 0 0 0 1 1 1
  line L53 (-56.1718, -23.8575) -> (-56.0153, -22.399)
  spline S159 degree 2 poles (-56.0153, -22.399) (-55.9836, -22.07) (-55.8692, -21.8598) knots 0 0 0 1 1 1
  spline S160 degree 2 poles (-55.8692, -21.8598) (-55.7549, -21.6496) (-55.549, -21.5378) knots 0 0 0 1 1 1
  spline S161 degree 2 poles (-55.549, -21.5378) (-55.3432, -21.4261) (-55.0353, -21.3927) knots 0 0 0 1 1 1
  line L54 (-55.0353, -21.3927) -> (-54.8084, -21.3681)
  line L55 (-55.0687, -23.3051) -> (-55.1356, -23.6816)
  line L56 (-55.1356, -23.6816) -> (-56.8967, -23.6816)
  line L57 (-56.8967, -23.6816) -> (-56.8298, -23.3051)
  line L58 (-56.8298, -23.3051) -> (-55.0687, -23.3051)
  line L59 (-43.2232, -17.443) -> (-44.3615, -19.943)
  line L60 (-44.3615, -19.943) -> (-44.935, -19.943)
  spline S162 degree 2 poles (-44.935, -19.943) (-44.9773, -19.7143) (-45.0133, -19.4627) knots 0 0 0 1 1 1
  spline S163 degree 2 poles (-45.0133, -19.4627) (-45.0494, -19.2111) (-45.0811, -18.9508) knots 0 0 0 1 1 1
  spline S164 degree 2 poles (-45.0811, -18.9508) (-45.1127, -18.6904) (-45.1382, -18.43) knots 0 0 0 1 1 1
  spline S165 degree 2 poles (-45.1382, -18.43) (-45.1637, -18.1696) (-45.1822, -17.9207) knots 0 0 0 1 1 1
  spline S166 degree 2 poles (-45.1822, -17.9207) (-45.2007, -17.6717) (-45.2112, -17.443) knots 0 0 0 1 1 1
  line L61 (-45.2112, -17.443) -> (-44.7767, -17.443)
  spline S167 degree 2 poles (-44.7767, -17.443) (-44.7732, -17.6242) (-44.7609, -17.8301) knots 0 0 0 1 1 1
  spline S168 degree 2 poles (-44.7609, -17.8301) (-44.7485, -18.0359) (-44.7318, -18.2514) knots 0 0 0 1 1 1
  spline S169 degree 2 poles (-44.7318, -18.2514) (-44.7151, -18.4669) (-44.694, -18.6842) knots 0 0 0 1 1 1
  spline S170 degree 2 poles (-44.694, -18.6842) (-44.6729, -18.9015) (-44.6509, -19.1073) knots 0 0 0 1 1 1
  spline S171 degree 2 poles (-44.6509, -19.1073) (-44.6289, -19.3132) (-44.606, -19.4961) knots 0 0 0 1 1 1
  line L62 (-44.606, -19.4961) -> (-44.5585, -19.4961)
  line L63 (-44.5585, -19.4961) -> (-43.6648, -17.443)
  line L64 (-43.6648, -17.443) -> (-43.2232, -17.443)
  line L65 (-43.6806, -17.9708) -> (-43.7457, -18.3614)
  line L66 (-43.7457, -18.3614) -> (-45.0124, -18.3614)
  line L67 (-45.0124, -18.3614) -> (-44.9474, -17.9708)
  line L68 (-44.9474, -17.9708) -> (-43.6806, -17.9708)
  line L69 (-45.4417, -16.6126) -> (-45.2517, -16.9838)
  spline S172 degree 2 poles (-45.2517, -16.9838) (-45.6581, -17.151) (-45.9607, -17.3682) knots 0 0 0 1 1 1
  spline S173 degree 2 poles (-45.9607, -17.3682) (-46.2633, -17.5855) (-46.4797, -17.867) knots 0 0 0 1 1 1
  spline S174 degree 2 poles (-46.4797, -17.867) (-46.6961, -18.1485) (-46.836, -18.5056) knots 0 0 0 1 1 1
  spline S175 degree 2 poles (-46.836, -18.5056) (-46.9759, -18.8628) (-47.055, -19.3079) knots 0 0 0 1 1 1
  line L70 (-47.055, -19.3079) -> (-47.4984, -19.3079)
  spline S176 degree 2 poles (-47.4984, -19.3079) (-47.3647, -18.613) (-47.106, -18.1001) knots 0 0 0 1 1 1
  spline S177 degree 2 poles (-47.106, -18.1001) (-46.8474, -17.5873) (-46.4384, -17.2249) knots 0 0 0 1 1 1
  spline S178 degree 2 poles (-46.4384, -17.2249) (-46.0293, -16.8624) (-45.4417, -16.6126) knots 0 0 0 1 1 1
  spline S179 degree 2 poles (-46.0311, -19.3431) (-46.2827, -18.3068) (-46.6996, -17.7755) knots 0 0 0 1 1 1
  line L71 (-46.6996, -17.7755) -> (-46.3302, -17.5433)
  spline S180 degree 2 poles (-46.3302, -17.5433) (-46.1085, -17.8741) (-45.9238, -18.313) knots 0 0 0 1 1 1
  spline S181 degree 2 poles (-45.9238, -18.313) (-45.739, -18.752) (-45.5825, -19.3079) knots 0 0 0 1 1 1
  line L72 (-45.5825, -19.3079) -> (-46.0311, -19.3431)
  line L73 (-48.2672, -19.3079) -> (-48.2443, -18.8276)
  line L74 (-48.2443, -18.8276) -> (-47.9998, -17.443)
  line L75 (-47.9998, -17.443) -> (-47.5635, -17.443)
  line L76 (-47.5635, -17.443) -> (-47.8942, -19.3079)
  line L77 (-47.8942, -19.3079) -> (-48.2672, -19.3079)
  line L78 (-48.2742, -17.443) -> (-48.5135, -18.803)
  spline S182 degree 2 poles (-48.5135, -18.803) (-48.5417, -18.9578) (-48.4273, -18.9578) knots 0 0 0 1 1 1
  spline S183 degree 2 poles (-48.4273, -18.9578) (-48.3446, -18.9578) (-48.2848, -18.8417) knots 0 0 0 1 1 1
  spline S184 degree 2 poles (-48.2848, -18.8417) (-48.225, -18.7256) (-48.1863, -18.5074) knots 0 0 0 1 1 1
  line L79 (-48.1863, -18.5074) -> (-48.2003, -19.0546)
  line L80 (-48.2003, -19.0546) -> (-48.2989, -19.0546)
  spline S185 degree 2 poles (-48.2989, -19.0546) (-48.3481, -19.2111) (-48.4291, -19.2771) knots 0 0 0 1 1 1
  spline S186 degree 2 poles (-48.4291, -19.2771) (-48.51, -19.3431) (-48.6314, -19.3431) knots 0 0 0 1 1 1
  spline S187 degree 2 poles (-48.6314, -19.3431) (-48.7809, -19.3431) (-48.839, -19.2252) knots 0 0 0 1 1 1
  spline S188 degree 2 poles (-48.839, -19.2252) (-48.897, -19.1073) (-48.8531, -18.8505) knots 0 0 0 1 1 1
  line L81 (-48.8531, -18.8505) -> (-48.6032, -17.443)
  line L82 (-48.6032, -17.443) -> (-48.2742, -17.443)
  line L83 (-49.5638, -18.8505) -> (-49.314, -17.443)
  line L84 (-49.314, -17.443) -> (-48.8759, -17.443)
  line L85 (-48.8759, -17.443) -> (-49.1169, -18.803)
  spline S189 degree 2 poles (-49.1169, -18.803) (-49.131, -18.8769) (-49.1108, -18.9173) knots 0 0 0 1 1 1
  spline S190 degree 2 poles (-49.1108, -18.9173) (-49.0906, -18.9578) (-49.0395, -18.9578) knots 0 0 0 1 1 1
  spline S191 degree 2 poles (-49.0395, -18.9578) (-48.9533, -18.9578) (-48.89, -18.8417) knots 0 0 0 1 1 1
  spline S192 degree 2 poles (-48.89, -18.8417) (-48.8267, -18.7256) (-48.7915, -18.5074) knots 0 0 0 1 1 1
  line L86 (-48.7915, -18.5074) -> (-48.7968, -19.0546)
  line L87 (-48.7968, -19.0546) -> (-48.9111, -19.0546)
  spline S193 degree 2 poles (-48.9111, -19.0546) (-48.9639, -19.2129) (-49.0563, -19.278) knots 0 0 0 1 1 1
  spline S194 degree 2 poles (-49.0563, -19.278) (-49.1486, -19.3431) (-49.2841, -19.3431) knots 0 0 0 1 1 1
  spline S195 degree 2 poles (-49.2841, -19.3431) (-49.6518, -19.3431) (-49.5638, -18.8505) knots 0 0 0 1 1 1
  spline S196 degree 2 poles (-50.2675, -17.4061) (-50.0142, -17.4061) (-49.8752, -17.5433) knots 0 0 0 1 1 1
  spline S197 degree 2 poles (-49.8752, -17.5433) (-49.7362, -17.6805) (-49.7362, -17.9304) knots 0 0 0 1 1 1
  spline S198 degree 2 poles (-49.7362, -17.9304) (-49.7362, -18.247) (-49.8752, -18.5048) knots 0 0 0 1 1 1
  spline S199 degree 2 poles (-49.8752, -18.5048) (-50.0142, -18.7625) (-50.2631, -18.9455) knots 0 0 0 1 1 1
  spline S200 degree 2 poles (-50.2631, -18.9455) (-50.5121, -19.1285) (-50.8472, -19.227) knots 0 0 0 1 1 1
  spline S201 degree 2 poles (-50.8472, -19.227) (-51.1824, -19.3255) (-51.5765, -19.3255) knots 0 0 0 1 1 1
  line L88 (-51.5765, -19.3255) -> (-51.6169, -19.3255)
  line L89 (-51.6169, -19.3255) -> (-51.39, -18.0254)
  spline S202 degree 2 poles (-51.39, -18.0254) (-51.3671, -17.8952) (-51.4129, -17.8424) knots 0 0 0 1 1 1
  spline S203 degree 2 poles (-51.4129, -17.8424) (-51.4586, -17.7896) (-51.6082, -17.7896) knots 0 0 0 1 1 1
  line L90 (-51.6082, -17.7896) -> (-51.6873, -17.7896)
  line L91 (-51.6873, -17.7896) -> (-51.624, -17.4254)
  line L92 (-51.624, -17.4254) -> (-51.4586, -17.4254)
  spline S204 degree 2 poles (-51.4586, -17.4254) (-51.2897, -17.4254) (-51.1921, -17.4615) knots 0 0 0 1 1 1
  spline S205 degree 2 poles (-51.1921, -17.4615) (-51.0944, -17.4976) (-51.0504, -17.5618) knots 0 0 0 1 1 1
  spline S206 degree 2 poles (-51.0504, -17.5618) (-51.0065, -17.626) (-51.0003, -17.7122) knots 0 0 0 1 1 1
  spline S207 degree 2 poles (-51.0003, -17.7122) (-50.9941, -17.7984) (-51.0082, -17.9022) knots 0 0 0 1 1 1
  line L93 (-51.0082, -17.9022) -> (-51.1191, -17.8565)
  line L94 (-51.1191, -17.8565) -> (-50.915, -17.8565)
  line L95 (-50.915, -17.8565) -> (-51.0188, -18.0394)
  spline S208 degree 2 poles (-51.0188, -18.0394) (-50.9255, -17.7386) (-50.7285, -17.5723) knots 0 0 0 1 1 1
  spline S209 degree 2 poles (-50.7285, -17.5723) (-50.5314, -17.4061) (-50.2675, -17.4061) knots 0 0 0 1 1 1
  spline S210 degree 2 poles (-50.3819, -17.8107) (-50.6229, -17.8107) (-50.8033, -18.021) knots 0 0 0 1 1 1
  spline S211 degree 2 poles (-50.8033, -18.021) (-50.9836, -18.2312) (-51.0504, -18.6165) knots 0 0 0 1 1 1
  line L96 (-51.0504, -18.6165) -> (-51.1419, -19.1267)
  line L97 (-51.1419, -19.1267) -> (-51.3003, -18.9209)
  spline S212 degree 2 poles (-51.3003, -18.9209) (-51.0645, -18.9103) (-50.8613, -18.8373) knots 0 0 0 1 1 1
  spline S213 degree 2 poles (-50.8613, -18.8373) (-50.6581, -18.7643) (-50.5051, -18.642) knots 0 0 0 1 1 1
  spline S214 degree 2 poles (-50.5051, -18.642) (-50.352, -18.5197) (-50.2658, -18.357) knots 0 0 0 1 1 1
  spline S215 degree 2 poles (-50.2658, -18.357) (-50.1796, -18.1942) (-50.1796, -18.006) knots 0 0 0 1 1 1
  spline S216 degree 2 poles (-50.1796, -18.006) (-50.1796, -17.9092) (-50.2315, -17.86) knots 0 0 0 1 1 1
  spline S217 degree 2 poles (-50.2315, -17.86) (-50.2834, -17.8107) (-50.3819, -17.8107) knots 0 0 0 1 1 1
  line L98 (-51.8844, -17.443) -> (-52.2134, -19.3079)
  line L99 (-52.2134, -19.3079) -> (-52.5881, -19.3079)
  line L100 (-52.5881, -19.3079) -> (-52.5758, -18.8628)
  line L101 (-52.5758, -18.8628) -> (-52.326, -17.443)
  line L102 (-52.326, -17.443) -> (-51.8844, -17.443)
  line L103 (-52.9963, -17.443) -> (-53.2021, -18.6147)
  spline S218 degree 2 poles (-53.2021, -18.6147) (-53.2302, -18.7748) (-53.1766, -18.8566) knots 0 0 0 1 1 1
  spline S219 degree 2 poles (-53.1766, -18.8566) (-53.1229, -18.9384) (-52.9963, -18.9384) knots 0 0 0 1 1 1
  spline S220 degree 2 poles (-52.9963, -18.9384) (-52.8784, -18.9384) (-52.7763, -18.8742) knots 0 0 0 1 1 1
  spline S221 degree 2 poles (-52.7763, -18.8742) (-52.6743, -18.81) (-52.5951, -18.6613) knots 0 0 0 1 1 1
  spline S222 degree 2 poles (-52.5951, -18.6613) (-52.516, -18.5127) (-52.4685, -18.2576) knots 0 0 0 1 1 1
  line L104 (-52.4685, -18.2576) -> (-52.5547, -18.9349)
  line L105 (-52.5547, -18.9349) -> (-52.6215, -18.9349)
  spline S223 degree 2 poles (-52.6215, -18.9349) (-52.6813, -19.1302) (-52.8256, -19.2366) knots 0 0 0 1 1 1
  spline S224 degree 2 poles (-52.8256, -19.2366) (-52.9699, -19.3431) (-53.1827, -19.3431) knots 0 0 0 1 1 1
  spline S225 degree 2 poles (-53.1827, -19.3431) (-53.4748, -19.3431) (-53.5918, -19.1592) knots 0 0 0 1 1 1
  spline S226 degree 2 poles (-53.5918, -19.1592) (-53.7088, -18.9754) (-53.6455, -18.6147) knots 0 0 0 1 1 1
  line L106 (-53.6455, -18.6147) -> (-53.4379, -17.443)
  line L107 (-53.4379, -17.443) -> (-52.9963, -17.443)
extrude "Extrude7" cut sketch "Sketch4" against normal blind 0.5 contours S0 S1 S2 S3 S4 S5 S6 S7 S8 S9 S10 S13 S14 S15 S16 S17 S18 S19 S20 S21 L9 S22 S27 L10 S28 S35 L11 | S8 L8 S9 S10 S11 S12 S13 S23 S24 S25 S26 S27 S28 S29 S30 S31 S32 S33 S34 S35 L11 L12 L13 L14 L16 S36 S37 | S8 L8 S9 S35 L11 | L18 L20 L21 L22 S43 L27 | L18 L19 L20 L22 L23 L24 L25 S38 S39 S40 L26 S41 S42 S43 | L18 L19 L20 L22 S43 L27 | S44 S45 S46 S47 S48 S49 S50 S51 | S60 S61 S62 S63 L28 S64 S65 S66 S67 S68 S69 L30 S70 S71 S72 S75 L32 L33 | L29 L30 S73 S74 S75 L33 L34 L35 S76 S77 L36 L37 L38 | S78 S79 L39 S80 S81 S82 S83 S84 S85 L40 S86 S87 S88 S89 S90 S91 L41 S92 S93 S94 S95 S96 S97 L42 S98 S99 S100 S101 | S102 S103 L43 S104 S105 S106 S107 S108 S109 L44 S110 S111 S112 S113 S114 S115 L45 S116 S117 S118 S119 S120 S121 L46 S122 S123 S124 S125 | S126 S127 L47 S128 S129 S130 S131 S132 S133 S134 S135 S136 S137 S138 S146 S147 | L49 L50 S148 S149 S150 L51 L53 S159 S160 S161 L54 L58 | L51 L53 L56 L58 | L53 L56 L57 L58 | L51 L55 L56 L58 | L51 S151 S152 S153 S154 L52 S155 S156 S157 S158 L53 L56 | L59 L60 S162 S163 S164 S165 S166 L61 S167 S168 S169 S170 S171 L62 L63 L64 L65 L66 L67 L68 | L63 L65 L66 L68 | S168 S169 L63 L66 L68 | S168 S169 L66 L67 L68 | L69 S172 S173 S174 S175 L70 S176 S177 S178 S179 L71 S180 | S173 S174 S179 S180 S181 L72 | L73 L74 L75 L76 L77 S184 L79 L80 | L73 L74 L78 S182 S183 S184 L80 S185 S186 S187 S188 L81 L82 S192 L86 L87 | S188 L81 L83 L84 L85 S189 S190 S191 S192 L87 S193 S194 S195 | S196 S197 S198 S199 S200 S201 L88 L89 S202 S203 L90 L91 L92 S204 S205 S206 S207 L94 S208 S209 | L98 L99 L100 L101 L102 S222 L104 L105 | L100 L101 L103 S218 S219 S220 S221 S222 L105 S223 S224 S225 S226 L106 L107 picked at (-40.4253, -22.9569) picked at (-41.777, -22.5978) picked at (-41.9688, -23.3202) picked at (-43.1435, -22.4594) picked at (-42.9781, -24.2633) picked at (-43.4003, -23.1685) picked at (-44.7373, -22.9759) picked at (-46.9621, -23.5816) picked at (-48.1734, -23.4159) picked at (-49.5157, -23.1209) picked at (-51.6269, -23.1209) picked at (-53.2742, -22.9925) picked at (-55.9345, -23.0031) picked at (-55.9936, -23.5561) picked at (-56.6265, -23.5561) picked at (-55.2934, -23.4306) picked at (-55.8897, -23.9214) picked at (-44.2219, -19.2669) picked at (-43.9016, -18.2312) picked at (-44.237, -18.101) picked at (-44.8972, -18.1945) picked at (-47.2865, -19.0338) picked at (-45.9147, -18.7572) picked at (-47.8813, -18.4194) picked at (-48.5264, -18.2511) picked at (-49.3316, -18.3655) picked at (-51.2469, -18.5209) picked at (-52.1887, -18.3362) picked at (-53.4285, -18.2242) bodies 2
